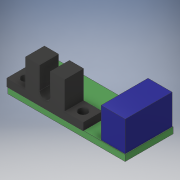
# Autodesk Inventor part: Endstop
Saved by Autodesk Inventor 2018 (Build 220112000, 112)
## iProperties
Created: 2012-11-09
Part Number: Endstop
Material: Generic
Document SubType Name: Modeling
Designer: Gabriel Smolnycki
Mass: 3.39359 g
Surface Area: 25.6627 cm^2
Volume: 3.39359 cm^3
Density: 1 g/cm^3
Appearance: Default
Author: Gabriel Smolnycki
Sending System: SolidWorks 2017
Last Author: Gabriel Smolnycki
Last Saved: 2017-09-14
Autodesk Inventor part; units mm, degrees
ref_plane "YZ Plane" through (0, 0, 0) normal (1, 0, 0) x (0, 1, 0)
ref_plane "XZ Plane" through (0, 0, 0) normal (0, 1, 0) x (-1, 0, 0)
ref_plane "Work Plane1" through (0, 0, 1.825) normal (0, 0, 1) x (1, 0, 0)
sketch "Sketch1" plane through (0, 0, 1.825) normal (0, 0, 1) x (1, 0, 0)
  line L0 (5.7, 2) -> (-19.7, 2)
  line L1 (5.7, 4.5) -> (5.7, 2)
  line L2 (-0.5, 13.7) -> (-5.2, 13.7)
  line L3 (-8.8, 6.3) -> (-8.8, 13.7)
  line L4 (-13.5, 4.5) -> (-19.7, 4.5)
  line L5 (5.7, 4.5) -> (-0.5, 4.5)
  line L6 (-5.2, 6.3) -> (-5.2, 13.7)
  line L7 (-8.8, 13.7) -> (-13.5, 13.7)
  line L8 (-19.7, 4.5) -> (-19.7, 2)
  line L9 (-0.5, 4.5) -> (-0.5, 13.7)
  arc A0 (-8.8, 6.3) -> (-5.2, 6.3) centre (-7, 6.3) ccw
  line L10 (-13.5, 4.5) -> (-13.5, 13.7)
  constraints: 22 end point, 6 vertical, 5 horizontal, 4 equal length, 2 point on circle, 1 centre point, 1 collinear
extrude "Extrusion3" add sketch "Sketch1" along normal blind 6.35
sketch "Sketch2" plane through (-19.7, 2, 1.825) normal (0, -1, 0) x (1, 0, 0)
  line L0 (0.2, 0) -> (0.2, 6.175)
  line L1 (0.2, 6.175) -> (25.4, 6.175)
  line L2 (25.4, 6.175) -> (39.2, 6.175)
  line L3 (39.2, 6.175) -> (39.2, -9.825)
  line L4 (39.2, -9.825) -> (0.2, -9.825)
  line L5 (0.2, -9.825) -> (0.2, 0)
  constraints: 12 end point, 3 horizontal, 3 vertical
extrude "Extrusion2" add sketch "Sketch2" along normal blind 2
hole "Hole2" at (-16.5, 0, 5) direction (0, 1, 0) diameter 3 depth 4.5
sketch "Sketch3" plane through (0, 0, 0) normal (0, 1, 0) x (-1, 0, 0)
  point P0 (16.5, 5)
hole "Hole1" at (2.5, 0, 5) direction (0, 1, 0) diameter 3 depth 4.5
sketch "Sketch5" plane through (-19.7, 2, 1.825) normal (0, 1, 0) x (1, 0, 0)
  line L0 (31, -5.975) -> (39, -5.975)
  line L1 (39, -5.975) -> (39, 9.625)
  line L2 (31, 9.625) -> (31, -5.975)
  line L3 (39, 9.625) -> (31, 9.625)
  constraints: 8 end point, 2 horizontal, 2 vertical
extrude "Extrusion1" add sketch "Sketch5" along normal blind 10
sketch "Sketch4" plane through (0, 0, 0) normal (0, 1, 0) x (-1, 0, 0)
  point P0 (-2.5, 5)
body "Solid3"
